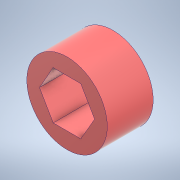
# Autodesk Inventor part: Churro Spacer
Saved by Autodesk Inventor 2020 (Build 240168000, 168)
## iProperties
Created: 2022-09-23
Part Number: Churro Spacer
Material: Generic
Document SubType Name: Modeling
Designer: Jason
Density: 1 g/cm^3
Appearance: Violet
Author: Jason
Autodesk Inventor part; units mm, degrees
ref_plane "YZ Plane" through (0, 0, 0) normal (1, 0, 0) x (0, 1, 0)
ref_plane "XZ Plane" through (0, 0, 0) normal (0, 1, 0) x (-1, 0, 0)
ref_plane "XY Plane" through (0, 0, 0) normal (0, 0, 1) x (1, 0, 0)
sketch "Sketch1" plane through (0, 0, 0) normal (0, 0, 1) x (1, 0, 0)
  circle A0 centre (0, 0) radius 11.1125
  line L0 (0, 0) -> (7.6256, 0)
  line L1 (-3.8526, 6.604) -> (3.8128, 6.604)
  line L2 (3.8128, 6.604) -> (7.6256, 0)
  line L3 (7.6256, 0) -> (3.8128, -6.604)
  line L4 (3.8128, -6.604) -> (-3.8128, -6.604)
  line L5 (-3.8128, -6.604) -> (-7.6056, -0.0348)
  line L6 (-7.6056, -0.0348) -> (-3.8526, 6.604)
  line L7 (0, 0) -> (0, 6.604)
  line L8 (0, 0) -> (0, -6.604)
  line L9 (0, 0) -> (-5.7192, 3.302)
  line L10 (0, 0) -> (5.7192, -3.302)
  line L11 (0, 0) -> (5.7192, 3.302)
  line L12 (0, 0) -> (-5.7192, -3.302)
  dimension "d0" = 22.225
  dimension "d16" = 13.208
  dimension "d17" = 13.208
  dimension "d19" = 6.604
  dimension "d20" = 6.604
  dimension "d21" = 6.604
  dimension "d22" = 6.604
  dimension "d23" = 60
  dimension "d24" = 60
  dimension "d25" = 6.604
  dimension "d26" = 6.604
  dimension "d27" = 60
  dimension "d28" = 60
  dimension "d29" = 0.52
  constraints: 26 end point, 3 midpoint, 2 point on line, 2 vertical, 1 centre point, 1 coincident, 1 horizontal, 1 parallel, 1 perpendicular
  measures "d0" diameter of A0
  measures "d16" distance between parallel lines of L5 L2
  measures "d17" distance between parallel lines of L4 L1
  measures "d19" distance of L0.start L7.end
  measures "d20" distance of L0.start L8.end
  measures "d21" distance of L0.start L9.end
  measures "d22" distance of L0.start L10.end
  measures "d23" angle of L7 L9
  measures "d24" angle of L8 L10
  measures "d25" distance of L0.start L11.end
  measures "d26" distance of L0.start L12.end
  measures "d27" angle of L8 L12
  measures "d28" angle of L7 L11
  measures "d29" angle of L3 L6
extrude "Extrusion1" add sketch "Sketch1" along normal blind 12.7
body "Solid1"
